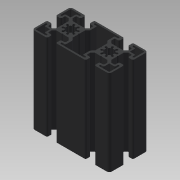
# Autodesk Inventor part: 45-4590
Saved by Autodesk Inventor 2013 (Build 170138000, 138)
## iProperties
Company: 80/20 Inc.
Created: 2014-04-23
Part Number: 45-4590
Material: Generic
Document SubType Name: Modeling
Designer: Ross Bowman
Density: 1 g/cm^3
Engineer: Ross Bowman
Catalog Web Link: 8020.net
Vendor: 80/20 Inc.
Material: 6105-T5 Aluminum
Author: Ross Bowman
Keywords: 80/20 , 8020 , T-Slot , Extrusion
Autodesk Inventor part; units mm, degrees
ref_plane "YZ Plane" through (0, 0, 0) normal (1, 0, 0) x (0, 1, 0)
ref_plane "XZ Plane" through (0, 0, 0) normal (0, 1, 0) x (-1, 0, 0)
ref_plane "XY Plane" through (0, 0, 0) normal (0, 0, 1) x (1, 0, 0)
sketch "Sketch1" plane through (0, 0, 0) normal (0, 0, 1) x (1, 0, 0)
  arc A0 (-28.343, 3.7238) -> (-29.7914, 3.2917) centre (-28.88, 2.8802) ccw
  line L0 (-26.716, 2.688) -> (-28.343, 3.7238)
  arc A1 (-25.1877, 4.2162) -> (-26.716, 2.688) centre (-22.5, 0) ccw
  line L1 (-26.2236, 5.8429) -> (-25.1877, 4.2162)
  arc A2 (-25.7915, 7.2915) -> (-26.2236, 5.8429) centre (-25.3801, 6.3801) ccw
  arc A3 (-25.3283, 7.4834) -> (-25.7915, 7.2915) centre (-22.5, 0) ccw
  arc A4 (-23.9985, 6.7647) -> (-25.3283, 7.4834) centre (-24.9747, 6.548) ccw
  line L2 (-23.5805, 4.8819) -> (-23.9985, 6.7647)
  arc A5 (-21.4192, 4.8818) -> (-23.5805, 4.8819) centre (-22.5, 0) ccw
  line L3 (-21.0014, 6.7645) -> (-21.4192, 4.8818)
  arc A6 (-19.6716, 7.4833) -> (-21.0014, 6.7645) centre (-20.0251, 6.5479) ccw
  arc A7 (-19.2083, 7.2914) -> (-19.6716, 7.4833) centre (-22.5, 0) ccw
  arc A8 (-18.7762, 5.843) -> (-19.2083, 7.2914) centre (-19.6198, 6.38) ccw
  line L4 (-19.812, 4.216) -> (-18.7762, 5.843)
  arc A9 (-18.2838, 2.6877) -> (-19.812, 4.216) centre (-22.5, 0) ccw
  line L5 (-16.6571, 3.7236) -> (-18.2838, 2.6877)
  arc A10 (-15.2085, 3.2915) -> (-16.6571, 3.7236) centre (-16.1199, 2.8801) ccw
  arc A11 (-15.0166, 2.8283) -> (-15.2085, 3.2915) centre (-22.5, 0) ccw
  arc A12 (-15.7353, 1.4985) -> (-15.0166, 2.8283) centre (-15.952, 2.4747) ccw
  line L6 (-17.6181, 1.0805) -> (-15.7353, 1.4985)
  arc A13 (-17.6182, -1.0808) -> (-17.6181, 1.0805) centre (-22.5, 0) ccw
  line L7 (-15.7355, -1.4986) -> (-17.6182, -1.0808)
  arc A14 (-15.0167, -2.8284) -> (-15.7355, -1.4986) centre (-15.9521, -2.4749) ccw
  arc A15 (-15.2086, -3.2917) -> (-15.0167, -2.8284) centre (-22.5, 0) ccw
  arc A16 (-16.657, -3.7238) -> (-15.2086, -3.2917) centre (-16.12, -2.8802) ccw
  line L8 (-18.284, -2.688) -> (-16.657, -3.7238)
  arc A17 (-19.8123, -4.2162) -> (-18.284, -2.688) centre (-22.5, 0) ccw
  line L9 (-18.7764, -5.8429) -> (-19.8123, -4.2162)
  arc A18 (-19.2085, -7.2915) -> (-18.7764, -5.8429) centre (-19.6199, -6.3801) ccw
  arc A19 (-19.6717, -7.4834) -> (-19.2085, -7.2915) centre (-22.5, 0) ccw
  arc A20 (-21.0015, -6.7647) -> (-19.6717, -7.4834) centre (-20.0253, -6.548) ccw
  line L10 (-21.4195, -4.8819) -> (-21.0015, -6.7647)
  arc A21 (-23.5808, -4.8818) -> (-21.4195, -4.8819) centre (-22.5, 0) ccw
  line L11 (-23.9986, -6.7645) -> (-23.5808, -4.8818)
  arc A22 (-25.3284, -7.4833) -> (-23.9986, -6.7645) centre (-24.9749, -6.5479) ccw
  arc A23 (-25.7917, -7.2914) -> (-25.3284, -7.4833) centre (-22.5, 0) ccw
  arc A24 (-26.2238, -5.843) -> (-25.7917, -7.2914) centre (-25.3802, -6.38) ccw
  line L12 (-25.188, -4.216) -> (-26.2238, -5.843)
  arc A25 (-26.7162, -2.6877) -> (-25.188, -4.216) centre (-22.5, 0) ccw
  line L13 (-28.3429, -3.7236) -> (-26.7162, -2.6877)
  arc A26 (-29.7915, -3.2915) -> (-28.3429, -3.7236) centre (-28.8801, -2.8801) ccw
  arc A27 (-29.9834, -2.8283) -> (-29.7915, -3.2915) centre (-22.5, 0) ccw
  arc A28 (-29.2647, -1.4985) -> (-29.9834, -2.8283) centre (-29.048, -2.4747) ccw
  line L14 (-27.3819, -1.0805) -> (-29.2647, -1.4985)
  arc A29 (-27.3818, 1.0808) -> (-27.3819, -1.0805) centre (-22.5, 0) ccw
  line L15 (-29.2645, 1.4986) -> (-27.3818, 1.0808)
  arc A30 (-29.9833, 2.8284) -> (-29.2645, 1.4986) centre (-29.0479, 2.4749) ccw
  arc A31 (-29.7914, 3.2917) -> (-29.9833, 2.8284) centre (-22.5, 0) ccw
  arc A32 (-31.5, 18.5) -> (-31.5, 20.5) centre (-31.5, 19.5) ccw
  line L16 (-33.5, 18.5) -> (-31.5, 18.5)
  arc A33 (-33.5, 18.5) -> (-34.5, 17.5) centre (-33.5, 17.5) ccw
  line L17 (-34.5, 12.38) -> (-34.5, 17.5)
  arc A34 (-34.88, 12) -> (-34.5, 12.38) centre (-34.88, 12.38) ccw
  line L18 (-40, 12) -> (-34.88, 12)
  arc A35 (-40, 12) -> (-41, 11) centre (-40, 11) ccw
  line L19 (-41, 9) -> (-41, 11)
  arc A36 (-43, 9) -> (-41, 9) centre (-42, 9) ccw
  line L20 (-43, 19.5) -> (-43, 9)
  arc A37 (-42, 20.5) -> (-43, 19.5) centre (-42, 19.5) ccw
  line L21 (-31.5, 20.5) -> (-42, 20.5)
  arc A38 (-41, -9) -> (-43, -9) centre (-42, -9) ccw
  line L22 (-41, -11) -> (-41, -9)
  arc A39 (-41, -11) -> (-40, -12) centre (-40, -11) ccw
  line L23 (-34.88, -12) -> (-40, -12)
  arc A40 (-34.5, -12.38) -> (-34.88, -12) centre (-34.88, -12.38) ccw
  line L24 (-34.5, -17.5) -> (-34.5, -12.38)
  arc A41 (-34.5, -17.5) -> (-33.5, -18.5) centre (-33.5, -17.5) ccw
  line L25 (-31.5, -18.5) -> (-33.5, -18.5)
  arc A42 (-31.5, -20.5) -> (-31.5, -18.5) centre (-31.5, -19.5) ccw
  line L26 (-42, -20.5) -> (-31.5, -20.5)
  arc A43 (-43, -19.5) -> (-42, -20.5) centre (-42, -19.5) ccw
  line L27 (-43, -9) -> (-43, -19.5)
  arc A44 (31.5, -18.5) -> (31.5, -20.5) centre (31.5, -19.5) ccw
  line L28 (33.5, -18.5) -> (31.5, -18.5)
  arc A45 (33.5, -18.5) -> (34.5, -17.5) centre (33.5, -17.5) ccw
  line L29 (34.5, -12.38) -> (34.5, -17.5)
  arc A46 (34.88, -12) -> (34.5, -12.38) centre (34.88, -12.38) ccw
  line L30 (40, -12) -> (34.88, -12)
  arc A47 (40, -12) -> (41, -11) centre (40, -11) ccw
  line L31 (41, -9) -> (41, -11)
  arc A48 (43, -9) -> (41, -9) centre (42, -9) ccw
  line L32 (43, -19.5) -> (43, -9)
  arc A49 (42, -20.5) -> (43, -19.5) centre (42, -19.5) ccw
  line L33 (31.5, -20.5) -> (42, -20.5)
  arc A50 (43, 19.5) -> (42, 20.5) centre (42, 19.5) ccw
  line L34 (43, 9) -> (43, 19.5)
  arc A51 (41, 9) -> (43, 9) centre (42, 9) ccw
  line L35 (41, 11) -> (41, 9)
  arc A52 (41, 11) -> (40, 12) centre (40, 11) ccw
  line L36 (34.88, 12) -> (40, 12)
  arc A53 (34.5, 12.38) -> (34.88, 12) centre (34.88, 12.38) ccw
  line L37 (34.5, 17.5) -> (34.5, 12.38)
  arc A54 (34.5, 17.5) -> (33.5, 18.5) centre (33.5, 17.5) ccw
  line L38 (31.5, 18.5) -> (33.5, 18.5)
  arc A55 (31.5, 20.5) -> (31.5, 18.5) centre (31.5, 19.5) ccw
  line L39 (42, 20.5) -> (31.5, 20.5)
  arc A56 (11.0487, -9.1603) -> (10.17, -11.2816) centre (13.17, -11.2816) ccw
  line L40 (10.17, -17.5) -> (10.17, -11.2816)
  arc A57 (10.17, -17.5) -> (11.17, -18.5) centre (11.17, -17.5) ccw
  line L41 (13.5, -18.5) -> (11.17, -18.5)
  arc A58 (13.5, -20.5) -> (13.5, -18.5) centre (13.5, -19.5) ccw
  line L42 (-13.5, -20.5) -> (13.5, -20.5)
  arc A59 (-13.5, -18.5) -> (-13.5, -20.5) centre (-13.5, -19.5) ccw
  line L43 (-11.17, -18.5) -> (-13.5, -18.5)
  arc A60 (-11.17, -18.5) -> (-10.17, -17.5) centre (-11.17, -17.5) ccw
  line L44 (-10.17, -11.2816) -> (-10.17, -17.5)
  arc A61 (-10.17, -11.2816) -> (-11.0487, -9.1603) centre (-13.17, -11.2816) ccw
  line L45 (-12.8887, -7.3203) -> (-11.0487, -9.1603)
  arc A62 (-13, -7.0516) -> (-12.8887, -7.3203) centre (-12.62, -7.0516) ccw
  line L46 (-13, -0.9) -> (-13, -7.0516)
  line L47 (-13.5196, 0) -> (-13, -0.9)
  line L48 (-13, 0.9) -> (-13.5196, 0)
  line L49 (-13, 7.0516) -> (-13, 0.9)
  arc A63 (-12.8887, 7.3203) -> (-13, 7.0516) centre (-12.62, 7.0516) ccw
  line L50 (-11.0487, 9.1603) -> (-12.8887, 7.3203)
  arc A64 (-11.0487, 9.1603) -> (-10.17, 11.2816) centre (-13.17, 11.2816) ccw
  line L51 (-10.17, 17.5) -> (-10.17, 11.2816)
  arc A65 (-10.17, 17.5) -> (-11.17, 18.5) centre (-11.17, 17.5) ccw
  line L52 (-13.5, 18.5) -> (-11.17, 18.5)
  arc A66 (-13.5, 20.5) -> (-13.5, 18.5) centre (-13.5, 19.5) ccw
  line L53 (13.5, 20.5) -> (-13.5, 20.5)
  arc A67 (13.5, 18.5) -> (13.5, 20.5) centre (13.5, 19.5) ccw
  line L54 (11.17, 18.5) -> (13.5, 18.5)
  arc A68 (11.17, 18.5) -> (10.17, 17.5) centre (11.17, 17.5) ccw
  line L55 (10.17, 11.2816) -> (10.17, 17.5)
  arc A69 (10.17, 11.2816) -> (11.0487, 9.1603) centre (13.17, 11.2816) ccw
  line L56 (12.8887, 7.3203) -> (11.0487, 9.1603)
  arc A70 (13, 7.0516) -> (12.8887, 7.3203) centre (12.62, 7.0516) ccw
  line L57 (13, 0.9) -> (13, 7.0516)
  line L58 (13.5196, 0) -> (13, 0.9)
  line L59 (13, -0.9) -> (13.5196, 0)
  line L60 (13, -7.0516) -> (13, -0.9)
  arc A71 (12.8887, -7.3203) -> (13, -7.0516) centre (12.62, -7.0516) ccw
  line L61 (11.0487, -9.1603) -> (12.8887, -7.3203)
  arc A72 (18.2838, -2.6877) -> (19.812, -4.216) centre (22.5, 0) ccw
  line L62 (16.6571, -3.7236) -> (18.2838, -2.6877)
  arc A73 (15.2085, -3.2915) -> (16.6571, -3.7236) centre (16.1199, -2.8801) ccw
  arc A74 (15.0166, -2.8283) -> (15.2085, -3.2915) centre (22.5, 0) ccw
  arc A75 (15.7353, -1.4985) -> (15.0166, -2.8283) centre (15.952, -2.4747) ccw
  line L63 (17.6181, -1.0805) -> (15.7353, -1.4985)
  arc A76 (17.6182, 1.0808) -> (17.6181, -1.0805) centre (22.5, 0) ccw
  line L64 (15.7355, 1.4986) -> (17.6182, 1.0808)
  arc A77 (15.0167, 2.8284) -> (15.7355, 1.4986) centre (15.9521, 2.4749) ccw
  arc A78 (15.2086, 3.2917) -> (15.0167, 2.8284) centre (22.5, 0) ccw
  arc A79 (16.657, 3.7238) -> (15.2086, 3.2917) centre (16.12, 2.8802) ccw
  line L65 (18.284, 2.688) -> (16.657, 3.7238)
  arc A80 (19.8123, 4.2162) -> (18.284, 2.688) centre (22.5, 0) ccw
  line L66 (18.7764, 5.8429) -> (19.8123, 4.2162)
  arc A81 (19.2085, 7.2915) -> (18.7764, 5.8429) centre (19.6199, 6.3801) ccw
  arc A82 (19.6717, 7.4834) -> (19.2085, 7.2915) centre (22.5, 0) ccw
  arc A83 (21.0015, 6.7647) -> (19.6717, 7.4834) centre (20.0253, 6.548) ccw
  line L67 (21.4195, 4.8819) -> (21.0015, 6.7647)
  arc A84 (23.5808, 4.8818) -> (21.4195, 4.8819) centre (22.5, 0) ccw
  line L68 (23.9986, 6.7645) -> (23.5808, 4.8818)
  arc A85 (25.3284, 7.4833) -> (23.9986, 6.7645) centre (24.9749, 6.5479) ccw
  arc A86 (25.7917, 7.2914) -> (25.3284, 7.4833) centre (22.5, 0) ccw
  arc A87 (26.2238, 5.843) -> (25.7917, 7.2914) centre (25.3802, 6.38) ccw
  line L69 (25.188, 4.216) -> (26.2238, 5.843)
  arc A88 (26.7162, 2.6877) -> (25.188, 4.216) centre (22.5, 0) ccw
  line L70 (28.3429, 3.7236) -> (26.7162, 2.6877)
  arc A89 (29.7915, 3.2915) -> (28.3429, 3.7236) centre (28.8801, 2.8801) ccw
  arc A90 (29.9834, 2.8283) -> (29.7915, 3.2915) centre (22.5, 0) ccw
  arc A91 (29.2647, 1.4985) -> (29.9834, 2.8283) centre (29.048, 2.4747) ccw
  line L71 (27.3819, 1.0805) -> (29.2647, 1.4985)
  arc A92 (27.3818, -1.0808) -> (27.3819, 1.0805) centre (22.5, 0) ccw
  line L72 (29.2645, -1.4986) -> (27.3818, -1.0808)
  arc A93 (29.9833, -2.8284) -> (29.2645, -1.4986) centre (29.0479, -2.4749) ccw
  arc A94 (29.7914, -3.2917) -> (29.9833, -2.8284) centre (22.5, 0) ccw
  arc A95 (28.343, -3.7238) -> (29.7914, -3.2917) centre (28.88, -2.8802) ccw
  line L73 (26.716, -2.688) -> (28.343, -3.7238)
  arc A96 (25.1877, -4.2162) -> (26.716, -2.688) centre (22.5, 0) ccw
  line L74 (26.2236, -5.8429) -> (25.1877, -4.2162)
  arc A97 (25.7915, -7.2915) -> (26.2236, -5.8429) centre (25.3801, -6.3801) ccw
  arc A98 (25.3283, -7.4834) -> (25.7915, -7.2915) centre (22.5, 0) ccw
  arc A99 (23.9985, -6.7647) -> (25.3283, -7.4834) centre (24.9747, -6.548) ccw
  line L75 (23.5805, -4.8819) -> (23.9985, -6.7647)
  arc A100 (21.4192, -4.8818) -> (23.5805, -4.8819) centre (22.5, 0) ccw
  line L76 (21.0014, -6.7645) -> (21.4192, -4.8818)
  arc A101 (19.6716, -7.4833) -> (21.0014, -6.7645) centre (20.0251, -6.5479) ccw
  arc A102 (19.2083, -7.2914) -> (19.6716, -7.4833) centre (22.5, 0) ccw
  arc A103 (18.7762, -5.843) -> (19.2083, -7.2914) centre (19.6198, -6.38) ccw
  line L77 (19.812, -4.216) -> (18.7762, -5.843)
  arc A104 (17.435, 20.98) -> (15.915, 22.5) centre (15.915, 20.98) ccw
  line L78 (15.915, 22.5) -> (-15.915, 22.5)
  arc A105 (-15.915, 22.5) -> (-17.435, 20.98) centre (-15.915, 20.98) ccw
  line L79 (-17.435, 20.98) -> (-17.435, 18.02)
  arc A106 (-17.435, 18.02) -> (-15.915, 16.5) centre (-15.915, 18.02) ccw
  line L80 (-15.915, 16.5) -> (-13.45, 16.5)
  arc A107 (-12.45, 15.5) -> (-13.45, 16.5) centre (-13.45, 15.5) ccw
  line L81 (-12.45, 15.5) -> (-12.45, 12.4984)
  arc A108 (-12.5613, 12.2297) -> (-12.45, 12.4984) centre (-12.83, 12.4984) ccw
  line L82 (-12.5613, 12.2297) -> (-15.1797, 9.6113)
  arc A109 (-15.4484, 9.5) -> (-15.1797, 9.6113) centre (-15.4484, 9.88) ccw
  line L83 (-15.4484, 9.5) -> (-21.6, 9.5)
  line L84 (-21.6, 9.5) -> (-22.5, 8.9849)
  line L85 (-22.5, 8.9849) -> (-23.4, 9.5)
  line L86 (-23.4, 9.5) -> (-29.5516, 9.5)
  arc A110 (-29.8203, 9.6113) -> (-29.5516, 9.5) centre (-29.5516, 9.88) ccw
  line L87 (-29.8203, 9.6113) -> (-32.4387, 12.2297)
  arc A111 (-32.55, 12.4984) -> (-32.4387, 12.2297) centre (-32.17, 12.4984) ccw
  line L88 (-32.55, 12.4984) -> (-32.55, 15.5)
  arc A112 (-31.55, 16.5) -> (-32.55, 15.5) centre (-31.55, 15.5) ccw
  line L89 (-31.55, 16.5) -> (-29.085, 16.5)
  arc A113 (-29.085, 16.5) -> (-27.565, 18.02) centre (-29.085, 18.02) ccw
  line L90 (-27.565, 18.02) -> (-27.565, 20.98)
  arc A114 (-27.565, 20.98) -> (-29.085, 22.5) centre (-29.085, 20.98) ccw
  line L91 (-29.085, 22.5) -> (-42, 22.5)
  arc A115 (-42, 22.5) -> (-45, 19.5) centre (-42, 19.5) ccw
  line L92 (-45, 19.5) -> (-45, 6.585)
  arc A116 (-45, 6.585) -> (-43.48, 5.065) centre (-43.48, 6.585) ccw
  line L93 (-43.48, 5.065) -> (-40.52, 5.065)
  arc A117 (-40.52, 5.065) -> (-39, 6.585) centre (-40.52, 6.585) ccw
  line L94 (-39, 6.585) -> (-39, 9.05)
  arc A118 (-38, 10.05) -> (-39, 9.05) centre (-38, 9.05) ccw
  line L95 (-38, 10.05) -> (-34.9984, 10.05)
  arc A119 (-34.7297, 9.9387) -> (-34.9984, 10.05) centre (-34.9984, 9.67) ccw
  line L96 (-34.7297, 9.9387) -> (-32.1113, 7.3203)
  arc A120 (-32, 7.0516) -> (-32.1113, 7.3203) centre (-32.38, 7.0516) ccw
  line L97 (-32, 7.0516) -> (-32, 0.9)
  line L98 (-32, 0.9) -> (-31.4804, 0)
  line L99 (-31.4804, 0) -> (-32, -0.9)
  line L100 (-32, -0.9) -> (-32, -7.0516)
  arc A121 (-32.1113, -7.3203) -> (-32, -7.0516) centre (-32.38, -7.0516) ccw
  line L101 (-32.1113, -7.3203) -> (-34.7297, -9.9387)
  arc A122 (-34.9984, -10.05) -> (-34.7297, -9.9387) centre (-34.9984, -9.67) ccw
  line L102 (-34.9984, -10.05) -> (-38, -10.05)
  arc A123 (-39, -9.05) -> (-38, -10.05) centre (-38, -9.05) ccw
  line L103 (-39, -9.05) -> (-39, -6.585)
  arc A124 (-39, -6.585) -> (-40.52, -5.065) centre (-40.52, -6.585) ccw
  line L104 (-40.52, -5.065) -> (-43.48, -5.065)
  arc A125 (-43.48, -5.065) -> (-45, -6.585) centre (-43.48, -6.585) ccw
  line L105 (-45, -6.585) -> (-45, -19.5)
  arc A126 (-45, -19.5) -> (-42, -22.5) centre (-42, -19.5) ccw
  line L106 (-42, -22.5) -> (-29.085, -22.5)
  arc A127 (-29.085, -22.5) -> (-27.565, -20.98) centre (-29.085, -20.98) ccw
  line L107 (-27.565, -20.98) -> (-27.565, -18.02)
  arc A128 (-27.565, -18.02) -> (-29.085, -16.5) centre (-29.085, -18.02) ccw
  line L108 (-29.085, -16.5) -> (-31.55, -16.5)
  arc A129 (-32.55, -15.5) -> (-31.55, -16.5) centre (-31.55, -15.5) ccw
  line L109 (-32.55, -15.5) -> (-32.55, -12.4984)
  arc A130 (-32.4387, -12.2297) -> (-32.55, -12.4984) centre (-32.17, -12.4984) ccw
  line L110 (-32.4387, -12.2297) -> (-29.8203, -9.6113)
  arc A131 (-29.5516, -9.5) -> (-29.8203, -9.6113) centre (-29.5516, -9.88) ccw
  line L111 (-29.5516, -9.5) -> (-23.4, -9.5)
  line L112 (-23.4, -9.5) -> (-22.5, -8.9849)
  line L113 (-22.5, -8.9849) -> (-21.6, -9.5)
  line L114 (-21.6, -9.5) -> (-15.4484, -9.5)
  arc A132 (-15.1797, -9.6113) -> (-15.4484, -9.5) centre (-15.4484, -9.88) ccw
  line L115 (-15.1797, -9.6113) -> (-12.5613, -12.2297)
  arc A133 (-12.45, -12.4984) -> (-12.5613, -12.2297) centre (-12.83, -12.4984) ccw
  line L116 (-12.45, -12.4984) -> (-12.45, -15.5)
  arc A134 (-13.45, -16.5) -> (-12.45, -15.5) centre (-13.45, -15.5) ccw
  line L117 (-13.45, -16.5) -> (-15.915, -16.5)
  arc A135 (-15.915, -16.5) -> (-17.435, -18.02) centre (-15.915, -18.02) ccw
  line L118 (-17.435, -18.02) -> (-17.435, -20.98)
  arc A136 (-17.435, -20.98) -> (-15.915, -22.5) centre (-15.915, -20.98) ccw
  line L119 (-15.915, -22.5) -> (15.915, -22.5)
  arc A137 (15.915, -22.5) -> (17.435, -20.98) centre (15.915, -20.98) ccw
  line L120 (17.435, -20.98) -> (17.435, -18.02)
  arc A138 (17.435, -18.02) -> (15.915, -16.5) centre (15.915, -18.02) ccw
  line L121 (15.915, -16.5) -> (13.45, -16.5)
  arc A139 (12.45, -15.5) -> (13.45, -16.5) centre (13.45, -15.5) ccw
  line L122 (12.45, -15.5) -> (12.45, -12.4984)
  arc A140 (12.5613, -12.2297) -> (12.45, -12.4984) centre (12.83, -12.4984) ccw
  line L123 (12.5613, -12.2297) -> (15.1797, -9.6113)
  arc A141 (15.4484, -9.5) -> (15.1797, -9.6113) centre (15.4484, -9.88) ccw
  line L124 (15.4484, -9.5) -> (21.6, -9.5)
  line L125 (21.6, -9.5) -> (22.5, -8.9849)
  line L126 (22.5, -8.9849) -> (23.4, -9.5)
  line L127 (23.4, -9.5) -> (29.5516, -9.5)
  arc A142 (29.8203, -9.6113) -> (29.5516, -9.5) centre (29.5516, -9.88) ccw
  line L128 (29.8203, -9.6113) -> (32.4387, -12.2297)
  arc A143 (32.55, -12.4984) -> (32.4387, -12.2297) centre (32.17, -12.4984) ccw
  line L129 (32.55, -12.4984) -> (32.55, -15.5)
  arc A144 (31.55, -16.5) -> (32.55, -15.5) centre (31.55, -15.5) ccw
  line L130 (31.55, -16.5) -> (29.085, -16.5)
  arc A145 (29.085, -16.5) -> (27.565, -18.02) centre (29.085, -18.02) ccw
  line L131 (27.565, -18.02) -> (27.565, -20.98)
  arc A146 (27.565, -20.98) -> (29.085, -22.5) centre (29.085, -20.98) ccw
  line L132 (29.085, -22.5) -> (42, -22.5)
  arc A147 (42, -22.5) -> (45, -19.5) centre (42, -19.5) ccw
  line L133 (45, -19.5) -> (45, -6.585)
  arc A148 (45, -6.585) -> (43.48, -5.065) centre (43.48, -6.585) ccw
  line L134 (43.48, -5.065) -> (40.52, -5.065)
  arc A149 (40.52, -5.065) -> (39, -6.585) centre (40.52, -6.585) ccw
  line L135 (39, -6.585) -> (39, -9.05)
  arc A150 (38, -10.05) -> (39, -9.05) centre (38, -9.05) ccw
  line L136 (38, -10.05) -> (34.9984, -10.05)
  arc A151 (34.7297, -9.9387) -> (34.9984, -10.05) centre (34.9984, -9.67) ccw
  line L137 (34.7297, -9.9387) -> (32.1113, -7.3203)
  arc A152 (32, -7.0516) -> (32.1113, -7.3203) centre (32.38, -7.0516) ccw
  line L138 (32, -7.0516) -> (32, -0.9)
  line L139 (32, -0.9) -> (31.4804, 0)
  line L140 (31.4804, 0) -> (32, 0.9)
  line L141 (32, 0.9) -> (32, 7.0516)
  arc A153 (32.1113, 7.3203) -> (32, 7.0516) centre (32.38, 7.0516) ccw
  line L142 (32.1113, 7.3203) -> (34.7297, 9.9387)
  arc A154 (34.9984, 10.05) -> (34.7297, 9.9387) centre (34.9984, 9.67) ccw
  line L143 (34.9984, 10.05) -> (38, 10.05)
  arc A155 (39, 9.05) -> (38, 10.05) centre (38, 9.05) ccw
  line L144 (39, 9.05) -> (39, 6.585)
  arc A156 (39, 6.585) -> (40.52, 5.065) centre (40.52, 6.585) ccw
  line L145 (40.52, 5.065) -> (43.48, 5.065)
  arc A157 (43.48, 5.065) -> (45, 6.585) centre (43.48, 6.585) ccw
  line L146 (45, 6.585) -> (45, 19.5)
  arc A158 (45, 19.5) -> (42, 22.5) centre (42, 19.5) ccw
  line L147 (42, 22.5) -> (29.085, 22.5)
  arc A159 (29.085, 22.5) -> (27.565, 20.98) centre (29.085, 20.98) ccw
  line L148 (27.565, 20.98) -> (27.565, 18.02)
  arc A160 (27.565, 18.02) -> (29.085, 16.5) centre (29.085, 18.02) ccw
  line L149 (29.085, 16.5) -> (31.55, 16.5)
  arc A161 (32.55, 15.5) -> (31.55, 16.5) centre (31.55, 15.5) ccw
  line L150 (32.55, 15.5) -> (32.55, 12.4984)
  arc A162 (32.4387, 12.2297) -> (32.55, 12.4984) centre (32.17, 12.4984) ccw
  line L151 (32.4387, 12.2297) -> (29.8203, 9.6113)
  arc A163 (29.5516, 9.5) -> (29.8203, 9.6113) centre (29.5516, 9.88) ccw
  line L152 (29.5516, 9.5) -> (23.4, 9.5)
  line L153 (23.4, 9.5) -> (22.5, 8.9849)
  line L154 (22.5, 8.9849) -> (21.6, 9.5)
  line L155 (21.6, 9.5) -> (15.4484, 9.5)
  arc A164 (15.1797, 9.6113) -> (15.4484, 9.5) centre (15.4484, 9.88) ccw
  line L156 (15.1797, 9.6113) -> (12.5613, 12.2297)
  arc A165 (12.45, 12.4984) -> (12.5613, 12.2297) centre (12.83, 12.4984) ccw
  line L157 (12.45, 12.4984) -> (12.45, 15.5)
  arc A166 (13.45, 16.5) -> (12.45, 15.5) centre (13.45, 15.5) ccw
  line L158 (13.45, 16.5) -> (15.915, 16.5)
  arc A167 (15.915, 16.5) -> (17.435, 18.02) centre (15.915, 18.02) ccw
  line L159 (17.435, 18.02) -> (17.435, 20.98)
  point P0 (0, 0)
  constraints: 336 point on circle, 320 end point, 168 centre point
extrude "Extrusion1" add sketch "Sketch1" against normal blind 100
body "Solid1"
